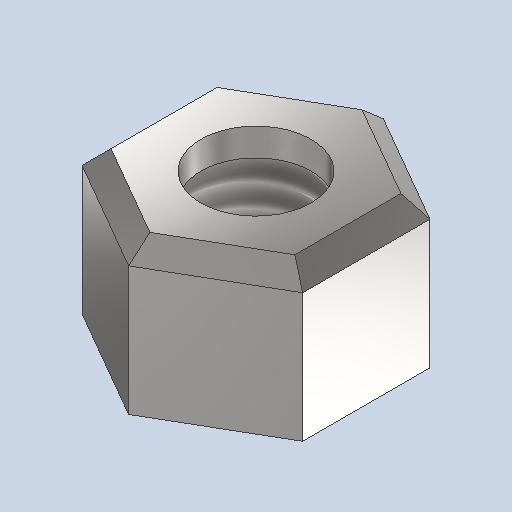
# Autodesk Inventor part: 50
Saved by Autodesk Inventor 2025.1 (Build 291241000, 241)
## iProperties
Created: 2024-09-18
Part Number: 50
Material: Steel, Alloy
Document SubType Name: Modeling
Designer: ffogue
Density: 7.73 g/cm^3
Appearance: Semi-Polished
Author: ffogue
Autodesk Inventor part; units mm, degrees
ref_plane "YZ Plane" through (0, 0, 0) normal (1, 0, 0) x (0, 1, 0)
ref_plane "XZ Plane" through (0, 0, 0) normal (0, 1, 0) x (-1, 0, 0)
ref_plane "XY Plane" through (0, 0, 0) normal (0, 0, 1) x (1, 0, 0)
sketch "Sketch1" plane through (0, 0, 0) normal (0, 0, 1) x (1, 0, 0)
  line L0 (0, 6.9282) -> (6, 3.4641)
  line L1 (6, 3.4641) -> (6, -3.4641)
  line L2 (6, -3.4641) -> (0, -6.9282)
  line L3 (0, -6.9282) -> (-6, -3.4641)
  line L4 (-6, -3.4641) -> (-6, 3.4641)
  line L5 (-6, 3.4641) -> (0, 6.9282)
  point P0 (0, 0)
  point P1 (0, 0)
  point P2 (-6, 0)
  dimension "d0" = 12
  constraints: 12 end point, 1 coincident, 1 horizontal alignment, 1 midpoint, 13 other
  measures "d0" distance between parallel lines of L1 L4
extrude "Extrusion1" add sketch "Sketch1" along normal blind 8
chamfer "Chamfer1" distance 1 angle 45 6 edges at (-3, 5.1962, 8) (3, 5.1962, 8) (6, 0, 8) (3, -5.1962, 8) (-3, -5.1962, 8) (-6, 0, 8)
sketch "Sketch2" plane through (0, 0, 8) normal (0, 0, 1) x (1, 0, 0)
  point P0 (0, 0)
  point P1 (0, 0)
  constraints: 1 coincident
hole "Hole1" at (0, 0, 8) direction (0, 0, -1) diameter 6 depth 1.5
sketch "Sketch3" plane through (0, 0, 0) normal (0, 0, -1) x (-1, 0, 0)
  point P0 (0, 0)
  point P1 (0, 0)
  constraints: 1 coincident
hole "Hole2" at (0, 0, 0) direction (0, 0, 1) diameter 6.647 depth 6.5 thread size "M8x1.25" class "6H" standard "ISO Metric profile"
body "Solid1"
